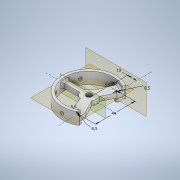
# Autodesk Inventor part: Verbindungsring_top
Saved by Autodesk Inventor 2020 (Build 240168000, 168)
## iProperties
Created: 2022-02-05
Part Number: Verbindungsring_top
Material: Generisch
Document SubType Name: Modeling
Designer: sp
Density: 1 g/cm^3
Appearance: Vorgabe
Author: sp
## iProperties of the stored document _3D-Druck.ipt
Created: 2022-05-01
Part Number: _3D-Druck
Material: Generisch
Document SubType Name: Modeling
Designer: sp
Density: 1 g/cm^3
Appearance: Vorgabe
Author: sp
Autodesk Inventor part; units mm, degrees
ref_plane "YZ Plane" through (0, 0, 0) normal (1, 0, 0) x (0, 1, 0)
sketch "Skizze5" plane through (0, 0, 0) normal (0, 1, 0) x (-1, 0, 0)
  circle A0 centre (0, 0) radius 27
  circle A1 centre (0, 0) radius 30
  dimension "d23" = 60
  dimension "d24" = 54
  constraints: 2 centre point, 2 coincident
  measures "d23" diameter of A1
  measures "d24" diameter of A0
extrude "Extrusion4" add sketch "Skizze5" along normal mid plane 2
sketch "Skizze6" plane through (0, 0, 0) normal (0, 1, 0) x (-1, 0, 0)
  circle A0 centre (0, 0) radius 27
  circle A1 centre (0, 0) radius 30
  dimension "d27" = 54
  dimension "d28" = 60
  constraints: 2 centre point, 2 coincident
  measures "d27" diameter of A0
  measures "d28" diameter of A1
extrude "Extrusion5" add sketch "Skizze6" along normal mid plane 13
ref_plane "Arbeitsebene5" through (0, 0, -30) normal (0, 0, 1) x (1, 0, 0)
sketch "Skizze7" plane through (0, 0, -30) normal (0, 0, 1) x (1, 0, 0)
  circle A0 centre (0, 0) radius 1.75
  line L0 (-34.5015, 0) -> (40.4508, 0) construction
  dimension "d33" = 3.5
  constraints: 2 end point, 1 centre point, 1 coincident, 1 horizontal, 1 point on line
  measures "d33" diameter of A0
extrude "Extrusion6" cut sketch "Skizze7" along normal blind 5
pattern_circular "Runde Anordnung2" count 3 over 360 about axis through (0, -10, 0) along (0, 1, 0) of "Extrusion6"
mirror "Spiegeln2" about plane through (0, 0, 0) normal (0, 0, 1) of "Extrusion6", "Runde Anordnung2"
sketch "Skizze21" plane through (0, 0, 0) normal (0, 1, 0) x (-1, 0, 0)
  circle A0 centre (0, 0) radius 30
  circle A1 centre (0, 0) radius 20.1927
  line L0 (-28.7132, 49.7328) -> (24.5245, -42.4776) construction
  line L1 (-23.684, -41.0219) -> (24.7886, 42.9352) construction
  line L2 (0, 59.1903) -> (0, -80.3627) construction
  line L3 (-24.7886, 42.9352) -> (20.7976, -36.0225)
  line L4 (11.9819, 20.7533) -> (-20.1927, -34.9748)
  line L5 (-6.029, 10.4426) -> (-6, -10.3923)
  line L6 (-6, -3) -> (-6, -26.3249) projected
  point P0 (-15, -25.9808)
  point P1 (-15, 25.9808)
  dimension "d96" = 120
  dimension "d97" = 30
  dimension "d127" = 40.3854
  dimension "d128" = 0.08
  constraints: 12 end point, 10 point on line, 2 centre point, 2 coincident, 1 vertical
  measures "d96" angle of L1 L0
  measures "d97" angle of L2 L1
  measures "d127" diameter of A1
  measures "d128" angle of L2 L5
extrude "Extrusion20" cut sketch "Skizze21" along normal mid plane 20 contours L3 A1 L4 A0 | L3 L5 L4 A1 picked at (-15.2279, -21.7631)
ref_plane "Arbeitsebene8" through (0, 0, 0) normal (0, 1, 0) x (-1, 0, 0)
sketch "Skizze23" plane through (0, 0, 0) normal (0, 1, 0) x (-1, 0, 0)
  line L0 (-16.5947, 0) -> (14.0429, 0) construction
  line L1 (0, 20.2219) -> (0, -26.4086) construction
  line L2 (0, 2.5) -> (27, 2.5)
  line L3 (27, 2.5) -> (27, -2.5)
  line L4 (27, -2.5) -> (0, -2.5)
  line L5 (0, -2.5) -> (0, 2.5)
  circle A0 centre (-10.0404, 21.9735) radius 5.5
  circle A1 centre (-10.0404, -22.0004) radius 5.5
  line L6 (-5.0542, 24.2947) -> (3.8228, 2.5)
  line L7 (3.8228, -2.5) -> (-4.9452, -24.0714)
  line L8 (-15.5404, -22.0004) -> (-4.9452, 0)
  line L9 (-15.2294, 20.1503) -> (-4.9452, 0)
  point P0 (0, 0)
  point P1 (-4.8514, 23.7968)
  point P2 (-14.5613, 18.8411)
  point P3 (-13.4695, -17.7002)
  dimension "d107" = 5
  dimension "d108" = 27
  dimension "d109" = 11
  dimension "d110" = 11
  constraints: 20 end point, 6 point on line, 4 point on circle, 2 centre point, 2 horizontal, 2 parallel, 1 perpendicular, 1 tangent, 1 vertical, 1 other
  measures "d107" distance between parallel lines of L4 L2
  measures "d108" distance of L3.end L4.end
  measures "d109" diameter of A0
  measures "d110" diameter of A1
extrude "Extrusion21" add sketch "Skizze23" along normal mid plane 5
sketch "Skizze22" plane through (0, 0, 0) normal (0, 1, 0) x (-1, 0, 0)
  line L0 (-10, 44.375) -> (-10, -60.1347) construction
  line L1 (-32.5458, 0) -> (48.0386, 0) construction
  circle A0 centre (-10, 22) radius 4.25
  circle A1 centre (-10, -22) radius 4.25
  circle A2 centre (-10, 22) radius 2.75
  circle A3 centre (-10, -22) radius 2.75
  point P0 (0, 0)
  dimension "d101" = 10
  dimension "d102" = 44
  dimension "d103" = 8.5
  dimension "d104" = 8.5
  dimension "d105" = 5.5
  dimension "d106" = 5.5
  constraints: 4 centre point, 4 end point, 3 point on line, 2 coincident, 1 horizontal, 1 symmetric about line, 1 vertical
  measures "d101" distance from line of point (0, 0) L0
  measures "d102" distance of A0.centre A1.centre
  measures "d103" diameter of A1
  measures "d104" diameter of A0
  measures "d105" diameter of A2
  measures "d106" diameter of A3
extrude "Extrusion22" cut sketch "Skizze22" against normal blind 10 contours A0 | A1 | A2 | A3
extrude "Extrusion23" add sketch "Skizze22" against normal blind 10 contours A2 | A3
fillet "Rundung10" radius 2 2 edges at (12.75, -10, 22) (12.75, -10, -22)
fillet "Rundung12" radius 2 2 edges at (6.5216, 0, 26.2006) (6.4968, 0, -26.2067)
fillet "Rundung13" radius 2 2 edges at (-26.884, 0, 2.5) (-26.884, 0, -2.5)
sketch "Skizze24" plane through (0, 0, 0) normal (0, 1, 0) x (-1, 0, 0)
  circle A0 centre (0, 0) radius 3.25
  dimension "d121" = 6.5
  constraints: 1 centre point, 1 coincident
  measures "d121" diameter of A0
extrude "Extrusion24" cut sketch "Skizze24" along normal mid plane 10
sketch "Skizze25" plane through (0, 0, 0) normal (0, 1, 0) x (-1, 0, 0)
  circle A0 centre (0, 0) radius 3.25
  circle A1 centre (0, 0) radius 8.2096
  constraints: 2 centre point, 2 coincident
extrude "Extrusion25" add sketch "Skizze25" along normal mid plane 5
fillet "Rundung14" radius 2 4 edges at (-26.8895, 2.5, 2.44) (-26.8895, 2.5, -2.44) (8.5929, 2.5, 25.5961) (8.5875, 2.5, -25.5979)
ref_plane "Arbeitsebene6" through (0, 0, 0) normal (0, 0, 1) x (1, 0, 0)
